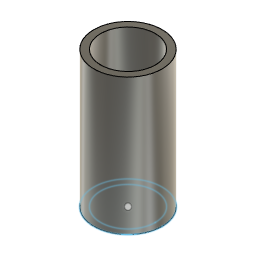
Razzetto v1 (Autodesk Fusion 360 design; units mm, degrees)
Autodesk Fusion 360 part; units mm, degrees
sketch "Schizzo1" plane through (0, 0, 0) normal (0, 0, 1) x (1, 0, 0)
  circle A0 centre (10, 10) radius 6.25
  circle A1 centre (10, 10) radius 5
  dimension "d1" = 12.5
  dimension "d4" = 10
  constraint concentric A0 A1
  measures "d1" diameter of A0
  measures "d4" diameter of A1
extrude "Estrusione1" add sketch "Schizzo1" along normal blind 25 contours A0 | A1
extrude "Estrusione3" cut sketch "Schizzo1" along normal blind 27 contours A1
extrude "Estrusione2" [suppressed]
